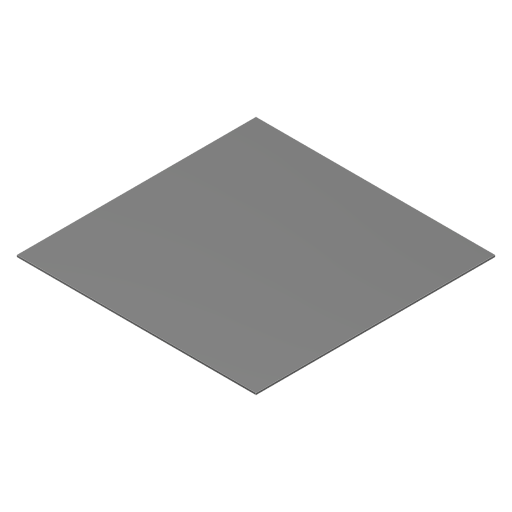
# Autodesk Inventor part: 42X42_BASE_PLATAFORMA
Saved by Autodesk Inventor 2024.2 (Build 282272000, 272)
## iProperties
Created: 2024-07-18
Part Number: 42X42_BASE_PLATAFORMA
Material: UHMW, Black
Document SubType Name: Modeling
Designer: jrcer
Density: 0.94 g/cm^3
Appearance: Smooth - Black
Author: jrcer
Autodesk Inventor part; units mm, degrees
ref_plane "YZ Plane" through (0, 0, 0) normal (1, 0, 0) x (0, 1, 0)
ref_plane "XZ Plane" through (0, 0, 0) normal (0, 1, 0) x (-1, 0, 0)
ref_plane "XY Plane" through (0, 0, 0) normal (0, 0, 1) x (1, 0, 0)
sketch "Sketch1" plane through (0, 0, 0) normal (0, 1, 0) x (-1, 0, 0)
  line L0 (210, 210) -> (-210, 210)
  line L1 (-210, 210) -> (-210, -210)
  line L2 (-210, -210) -> (210, -210)
  line L3 (210, -210) -> (210, 210)
  line L4 (210, 210) -> (-210, -210) construction
  line L5 (-210, 210) -> (210, -210) construction
  point P0 (0, 0)
  dimension "d0" = 420
  dimension "d1" = 420
  constraints: 12 end point, 2 midpoint, 2 parallel, 1 horizontal, 1 perpendicular
  measures "d0" distance of L2.end L1.end
  measures "d1" distance of L1.end L0.end
extrude "Extrusion1" add sketch "Sketch1" along normal blind 3.25
sketch "Sketch3" plane through (0, 3.25, 0) normal (0, 1, 0) x (1, 0, 0)
  line L0 (210, -210) -> (210, 210) construction
  line L1 (210, 210) -> (-210, 210) construction
  line L2 (-210, 210) -> (-210, -210) construction
  line L3 (-210, -210) -> (210, -210) construction
  line L4 (-200, 200) -> (200, 200)
  line L5 (200, 200) -> (200, -200)
  line L6 (200, -200) -> (-200, -200)
  line L7 (-200, -200) -> (-200, 200)
  line L8 (-200, 200) -> (200, -200) construction
  line L9 (200, 200) -> (-200, -200) construction
  point P0 (0, 0)
  dimension "d9" = 400
  dimension "d10" = 400
  constraints: 12 end point, 2 midpoint, 2 parallel, 1 horizontal, 1 perpendicular
  measures "d9" distance of L5.end L6.end
  measures "d10" distance of L4.end L5.end
body "Solid1"
